Autodesk Fusion 360 part; units mm, degrees
(part 2 of 2)
sketch "Sketch5" plane through (0, 0, 32) normal (0, 0, 1) x (-1, 0, 0)
  line L0 (-236, -90) -> (0, -90)
  line L1 (0, -90) -> (0, -50)
  line L2 (0, -50) -> (-236, -50)
  line L3 (-236, -50) -> (-236, -90)
  line L4 (-4, -87) -> (-4, -53)
  line L5 (-108, -90) -> (-118, -90)
  line L6 (-4, -53) -> (-10, -53)
  line L7 (0, -90) -> (-10, -90)
  line L8 (0, -50) -> (0, -90)
  line L9 (-114, -87) -> (-114, -53)
  line L10 (0, -90) -> (-10, -90)
  line L11 (-118, -90) -> (-118, -50)
  line L12 (-10, -90) -> (-108, -90)
  line L13 (-10, -90) -> (-10, -50)
  line L14 (-108, -87) -> (-114, -87)
  line L15 (-4, -53) -> (-10, -53)
  line L16 (-10, -87) -> (-4, -87)
  line L17 (-10, -53) -> (-10, -87)
  line L18 (-108, -50) -> (-108, -90)
  line L19 (-10, -53) -> (-10, -87)
  line L20 (-118, -50) -> (-108, -50)
  line L21 (-108, -50) -> (-10, -50)
  line L22 (-10, -87) -> (-4, -87)
  line L23 (-108, -90) -> (-108, -50)
  line L24 (-114, -53) -> (-108, -53)
  line L25 (0, -50) -> (0, -90)
  line L26 (-10, -50) -> (0, -50)
  line L27 (-4, -87) -> (-4, -53)
  line L28 (-108, -53) -> (-108, -87)
  line L29 (-10, -50) -> (0, -50)
  line L30 (-10, -90) -> (-10, -50)
  line L31 (-10, -50) -> (-10, -90)
  line L32 (-122, -87) -> (-122, -53)
  line L33 (-226, -90) -> (-236, -90)
  line L34 (-122, -53) -> (-128, -53)
  line L35 (-118, -90) -> (-128, -90)
  line L36 (-118, -50) -> (-118, -90)
  line L37 (-232, -87) -> (-232, -53)
  line L38 (-118, -90) -> (-128, -90)
  line L39 (-236, -90) -> (-236, -50)
  line L40 (-128, -90) -> (-226, -90)
  line L41 (-128, -90) -> (-128, -50)
  line L42 (-226, -87) -> (-232, -87)
  line L43 (-122, -53) -> (-128, -53)
  line L44 (-128, -87) -> (-122, -87)
  line L45 (-128, -53) -> (-128, -87)
  line L46 (-226, -50) -> (-226, -90)
  line L47 (-128, -53) -> (-128, -87)
  line L48 (-236, -50) -> (-226, -50)
  line L49 (-226, -50) -> (-128, -50)
  line L50 (-128, -87) -> (-122, -87)
  line L51 (-226, -90) -> (-226, -50)
  line L52 (-232, -53) -> (-226, -53)
  line L53 (-118, -50) -> (-118, -90)
  line L54 (-128, -50) -> (-118, -50)
  line L55 (-122, -87) -> (-122, -53)
  line L56 (-226, -53) -> (-226, -87)
  line L57 (-128, -50) -> (-118, -50)
  line L58 (-128, -90) -> (-128, -50)
  line L59 (-128, -50) -> (-128, -90)
  line L60 (-4, -177) -> (-4, -143)
  line L61 (-108, -180) -> (-118, -180)
  line L62 (-4, -143) -> (-10, -143)
  line L63 (0, -180) -> (-10, -180)
  line L64 (0, -140) -> (0, -180)
  line L65 (-114, -177) -> (-114, -143)
  line L66 (0, -180) -> (-10, -180)
  line L67 (-118, -180) -> (-118, -140)
  line L68 (-10, -180) -> (-108, -180)
  line L69 (-10, -180) -> (-10, -140)
  line L70 (-108, -177) -> (-114, -177)
  line L71 (-4, -143) -> (-10, -143)
  line L72 (-10, -177) -> (-4, -177)
  line L73 (-10, -143) -> (-10, -177)
  line L74 (-108, -140) -> (-108, -180)
  line L75 (-10, -143) -> (-10, -177)
  line L76 (-118, -140) -> (-108, -140)
  line L77 (-108, -140) -> (-10, -140)
  line L78 (-10, -177) -> (-4, -177)
  line L79 (-108, -180) -> (-108, -140)
  line L80 (-114, -143) -> (-108, -143)
  line L81 (0, -140) -> (0, -180)
  line L82 (-10, -140) -> (0, -140)
  line L83 (-4, -177) -> (-4, -143)
  line L84 (-108, -143) -> (-108, -177)
  line L85 (-10, -140) -> (0, -140)
  line L86 (-10, -180) -> (-10, -140)
  line L87 (-10, -140) -> (-10, -180)
  line L88 (-122, -177) -> (-122, -143)
  line L89 (-226, -180) -> (-236, -180)
  line L90 (-122, -143) -> (-128, -143)
  line L91 (-118, -180) -> (-128, -180)
  line L92 (-118, -140) -> (-118, -180)
  line L93 (-232, -177) -> (-232, -143)
  line L94 (-118, -180) -> (-128, -180)
  line L95 (-236, -180) -> (-236, -140)
  line L96 (-128, -180) -> (-226, -180)
  line L97 (-128, -180) -> (-128, -140)
  line L98 (-226, -177) -> (-232, -177)
  line L99 (-122, -143) -> (-128, -143)
  line L100 (-128, -177) -> (-122, -177)
  line L101 (-128, -143) -> (-128, -177)
  line L102 (-226, -140) -> (-226, -180)
  line L103 (-128, -143) -> (-128, -177)
  line L104 (-236, -140) -> (-226, -140)
  line L105 (-226, -140) -> (-128, -140)
  line L106 (-128, -177) -> (-122, -177)
  line L107 (-226, -180) -> (-226, -140)
  line L108 (-232, -143) -> (-226, -143)
  line L109 (-118, -140) -> (-118, -180)
  line L110 (-128, -140) -> (-118, -140)
  line L111 (-122, -177) -> (-122, -143)
  line L112 (-226, -143) -> (-226, -177)
  line L113 (-128, -140) -> (-118, -140)
  line L114 (-128, -180) -> (-128, -140)
  line L115 (-128, -140) -> (-128, -180)
  line L116 (-4, -87) -> (-4, -53)
  line L117 (-108, -90) -> (-118, -90)
  line L118 (-4, -53) -> (-10, -53)
  line L119 (0, -90) -> (-10, -90)
  line L120 (0, -50) -> (0, -90)
  line L121 (-114, -87) -> (-114, -53)
  line L122 (0, -90) -> (-10, -90)
  line L123 (-118, -90) -> (-118, -50)
  line L124 (-10, -90) -> (-108, -90)
  line L125 (-10, -90) -> (-10, -50)
  line L126 (-108, -87) -> (-114, -87)
  line L127 (-4, -53) -> (-10, -53)
  line L128 (-10, -87) -> (-4, -87)
  line L129 (-10, -53) -> (-10, -87)
  line L130 (-108, -50) -> (-108, -90)
  line L131 (-10, -53) -> (-10, -87)
  line L132 (-118, -50) -> (-108, -50)
  line L133 (-108, -50) -> (-10, -50)
  line L134 (-10, -87) -> (-4, -87)
  line L135 (-108, -90) -> (-108, -50)
  line L136 (-114, -53) -> (-108, -53)
  line L137 (0, -50) -> (0, -90)
  line L138 (-10, -50) -> (0, -50)
  line L139 (-4, -87) -> (-4, -53)
  line L140 (-108, -53) -> (-108, -87)
  line L141 (-10, -50) -> (0, -50)
  line L142 (-10, -90) -> (-10, -50)
  line L143 (-10, -50) -> (-10, -90)
  line L144 (-128, -267) -> (-122, -267)
  line L145 (-10, -230) -> (0, -230)
  line L146 (0, -270) -> (-10, -270)
  line L147 (-128, -230) -> (-128, -270)
  line L148 (-118, -270) -> (-118, -230)
  line L149 (-226, -233) -> (-226, -267)
  line L150 (0, -230) -> (0, -270)
  line L151 (-108, -270) -> (-118, -270)
  line L152 (-118, -270) -> (-128, -270)
  line L153 (-226, -270) -> (-226, -230)
  line L154 (-118, -230) -> (-108, -230)
  line L155 (0, -230) -> (0, -270)
  line L156 (-128, -230) -> (-118, -230)
  line L157 (-10, -230) -> (-10, -270)
  line L158 (-118, -230) -> (-118, -270)
  line L159 (-10, -270) -> (-108, -270)
  line L160 (-10, -267) -> (-4, -267)
  line L161 (-10, -233) -> (-10, -267)
  line L162 (-128, -230) -> (-118, -230)
  line L163 (-10, -270) -> (-10, -230)
  line L164 (-236, -270) -> (-236, -230)
  line L165 (-128, -270) -> (-128, -230)
  line L166 (-122, -233) -> (-128, -233)
  line L167 (-10, -267) -> (-4, -267)
  line L168 (-122, -267) -> (-122, -233)
  line L169 (-10, -233) -> (-10, -267)
  line L170 (-10, -270) -> (-10, -230)
  line L171 (-236, -230) -> (-226, -230)
  line L172 (-128, -270) -> (-128, -230)
  line L173 (-128, -233) -> (-128, -267)
  line L174 (-226, -267) -> (-232, -267)
  line L175 (-108, -233) -> (-108, -267)
  line L176 (-128, -233) -> (-128, -267)
  line L177 (-122, -267) -> (-122, -233)
  line L178 (-118, -270) -> (-128, -270)
  line L179 (-226, -230) -> (-128, -230)
  line L180 (-4, -233) -> (-10, -233)
  line L181 (-10, -230) -> (0, -230)
  line L182 (-108, -230) -> (-10, -230)
  line L183 (-4, -233) -> (-10, -233)
  line L184 (0, -270) -> (-10, -270)
  line L185 (-108, -267) -> (-114, -267)
  line L186 (-128, -270) -> (-226, -270)
  line L187 (-4, -267) -> (-4, -233)
  line L188 (-128, -267) -> (-122, -267)
  line L189 (-114, -233) -> (-108, -233)
  line L190 (-232, -267) -> (-232, -233)
  line L191 (-114, -267) -> (-114, -233)
  line L192 (-226, -230) -> (-226, -270)
  line L193 (-232, -233) -> (-226, -233)
  line L194 (-108, -270) -> (-108, -230)
  line L195 (-226, -270) -> (-236, -270)
  line L196 (-122, -233) -> (-128, -233)
  line L197 (-108, -230) -> (-108, -270)
  line L198 (-4, -267) -> (-4, -233)
  line L199 (-118, -230) -> (-118, -270)
  dimension "d47" = 10
  dimension "d48" = 40
  dimension "d49" = 3
  dimension "d50" = 4
  dimension "d51" = 3
  dimension "d52" = 10
  dimension "d53" = 40
  dimension "d54" = 3
  dimension "d55" = 4
  dimension "d56" = 3
  dimension "d57" = 10
  dimension "d58" = 40
  dimension "d59" = 98
  dimension "d60" = 3
  dimension "d61" = 3
  dimension "d62" = 4
  dimension "d63" = 10
  dimension "d64" = 40
  dimension "d65" = 3
  dimension "d66" = 4
  dimension "d67" = 3
  dimension "d68" = 10
  dimension "d69" = 40
  dimension "d70" = 3
  dimension "d71" = 4
  dimension "d72" = 3
  dimension "d73" = 10
  dimension "d74" = 40
  dimension "d75" = 98
  dimension "d76" = 3
  dimension "d77" = 3
  dimension "d78" = 4
  dimension "d79" = 10
  dimension "d80" = 40
  dimension "d81" = 3
  dimension "d82" = 4
  dimension "d83" = 3
  dimension "d84" = 10
  dimension "d85" = 40
  dimension "d86" = 3
  dimension "d87" = 4
  dimension "d88" = 3
  dimension "d89" = 10
  dimension "d90" = 40
  dimension "d91" = 98
  dimension "d92" = 3
  dimension "d93" = 3
  dimension "d94" = 4
  dimension "d95" = 10
  dimension "d96" = 40
  dimension "d97" = 3
  dimension "d98" = 4
  dimension "d99" = 3
  dimension "d100" = 10
  dimension "d101" = 40
  dimension "d102" = 3
  dimension "d103" = 4
  dimension "d104" = 3
  dimension "d105" = 10
  dimension "d106" = 40
  dimension "d107" = 98
  dimension "d108" = 3
  dimension "d109" = 3
  dimension "d110" = 4
  dimension "d111" = 10
  dimension "d112" = 40
  dimension "d113" = 3
  dimension "d114" = 4
  dimension "d115" = 3
  dimension "d116" = 10
  dimension "d117" = 40
  dimension "d118" = 3
  dimension "d119" = 4
  dimension "d120" = 3
  dimension "d121" = 10
  dimension "d122" = 40
  dimension "d123" = 98
  dimension "d124" = 3
  dimension "d125" = 3
  dimension "d126" = 4
  dimension "d127" = 10
  dimension "d128" = 40
  dimension "d129" = 3
  dimension "d130" = 4
  dimension "d131" = 3
  dimension "d132" = 10
  dimension "d133" = 40
  dimension "d134" = 3
  dimension "d135" = 4
  dimension "d136" = 3
  dimension "d137" = 10
  dimension "d138" = 40
  dimension "d139" = 98
  dimension "d140" = 3
  dimension "d141" = 3
  dimension "d142" = 4
  dimension "d143" = 10
  dimension "d144" = 40
  dimension "d145" = 3
  dimension "d146" = 4
  dimension "d147" = 3
  dimension "d148" = 10
  dimension "d149" = 40
  dimension "d150" = 3
  dimension "d151" = 4
  dimension "d152" = 3
  dimension "d153" = 10
  dimension "d154" = 40
  dimension "d155" = 98
  dimension "d156" = 3
  dimension "d157" = 3
  dimension "d158" = 4
  constraint horizontal L10
  constraint vertical L13
  constraint horizontal L26
  constraint vertical L8
  constraint horizontal L22
  constraint vertical L4
  constraint horizontal L6
  constraint vertical L17
  constraint coincident L16.start L13
  constraint horizontal L7
  constraint vertical L30
  constraint horizontal L29
  constraint vertical L25
  constraint horizontal L16
  constraint vertical L27
  constraint horizontal L15
  constraint vertical L19
  constraint coincident L16.start L30
  constraint horizontal L5
  constraint vertical L11
  constraint horizontal L20
  constraint vertical L18
  constraint horizontal L14
  constraint vertical L9
  constraint horizontal L24
  constraint vertical L28
  constraint coincident L14.start L18
  constraint horizontal L12
  constraint vertical L23
  constraint horizontal L21
  constraint vertical L31
  constraint horizontal L38
  constraint vertical L41
  constraint horizontal L54
  constraint vertical L36
  constraint horizontal L50
  constraint vertical L32
  constraint horizontal L34
  constraint vertical L45
  constraint coincident L44.start L41
  constraint horizontal L35
  constraint vertical L58
  constraint horizontal L57
  constraint vertical L53
  constraint horizontal L44
  constraint vertical L55
  constraint horizontal L43
  constraint vertical L47
  constraint coincident L44.start L58
  constraint horizontal L33
  constraint vertical L39
  constraint horizontal L48
  constraint vertical L46
  constraint horizontal L42
  constraint vertical L37
  constraint horizontal L52
  constraint vertical L56
  constraint coincident L42.start L46
  constraint horizontal L40
  constraint vertical L51
  constraint horizontal L49
  constraint vertical L59
  constraint horizontal L66
  constraint vertical L69
  constraint horizontal L82
  constraint vertical L64
  constraint horizontal L78
  constraint vertical L60
  constraint horizontal L62
  constraint vertical L73
  constraint coincident L72.start L69
  constraint horizontal L63
  constraint vertical L86
  constraint horizontal L85
  constraint vertical L81
  constraint horizontal L72
  constraint vertical L83
  constraint horizontal L71
  constraint vertical L75
  constraint coincident L72.start L86
  constraint horizontal L61
  constraint vertical L67
  constraint horizontal L76
  constraint vertical L74
  constraint horizontal L70
  constraint vertical L65
  constraint horizontal L80
  constraint vertical L84
  constraint coincident L70.start L74
  constraint horizontal L68
  constraint vertical L79
  constraint horizontal L77
  constraint vertical L87
  constraint horizontal L94
  constraint vertical L97
  constraint horizontal L110
  constraint vertical L92
  constraint horizontal L106
  constraint vertical L88
  constraint horizontal L90
  constraint vertical L101
  constraint coincident L100.start L97
  constraint horizontal L91
  constraint vertical L114
  constraint horizontal L113
  constraint vertical L109
  constraint horizontal L100
  constraint vertical L111
  constraint horizontal L99
  constraint vertical L103
  constraint coincident L100.start L114
  constraint horizontal L89
  constraint vertical L95
  constraint horizontal L104
  constraint vertical L102
  constraint horizontal L98
  constraint vertical L93
  constraint horizontal L108
  constraint vertical L112
  constraint coincident L98.start L102
  constraint horizontal L96
  constraint vertical L107
  constraint horizontal L105
  constraint vertical L115
  constraint horizontal L122
  constraint vertical L125
  constraint horizontal L138
  constraint vertical L120
  constraint horizontal L134
  constraint vertical L116
  constraint horizontal L118
  constraint vertical L129
  constraint coincident L16.start L125
  constraint horizontal L119
  constraint vertical L142
  constraint horizontal L141
  constraint vertical L137
  constraint horizontal L128
  constraint vertical L139
  constraint horizontal L127
  constraint vertical L131
  constraint coincident L16.start L142
  constraint horizontal L117
  constraint vertical L123
  constraint horizontal L132
  constraint vertical L130
  constraint horizontal L126
  constraint vertical L121
  constraint horizontal L136
  constraint vertical L140
  constraint coincident L14.start L130
  constraint horizontal L124
  constraint vertical L135
  constraint horizontal L133
  constraint vertical L143
  constraint horizontal L184
  constraint vertical L163
  constraint horizontal L145
  constraint vertical L155
  constraint horizontal L160
  constraint vertical L187
  constraint horizontal L180
  constraint vertical L161
  constraint coincident L160.start L163
  constraint horizontal L146
  constraint vertical L170
  constraint horizontal L181
  constraint vertical L150
  constraint horizontal L167
  constraint vertical L198
  constraint horizontal L183
  constraint vertical L169
  constraint coincident L160.start L170
  constraint horizontal L151
  constraint vertical L148
  constraint horizontal L154
  constraint vertical L197
  constraint horizontal L185
  constraint vertical L191
  constraint horizontal L189
  constraint vertical L175
  constraint coincident L175.end L197
  constraint horizontal L159
  constraint vertical L194
  constraint horizontal L182
  constraint vertical L157
  constraint horizontal L178
  constraint vertical L165
  constraint horizontal L162
  constraint vertical L158
  constraint horizontal L188
  constraint vertical L168
  constraint horizontal L196
  constraint vertical L176
  constraint coincident L144.start L165
  constraint horizontal L152
  constraint vertical L172
  constraint horizontal L156
  constraint vertical L199
  constraint horizontal L144
  constraint vertical L177
  constraint horizontal L166
  constraint vertical L173
  constraint coincident L144.start L172
  constraint horizontal L195
  constraint vertical L164
  constraint horizontal L171
  constraint vertical L192
  constraint horizontal L174
  constraint vertical L190
  constraint horizontal L193
  constraint vertical L149
  constraint coincident L149.end L192
  constraint horizontal L186
  constraint vertical L153
  constraint horizontal L179
  constraint vertical L147
  measures "d47" distance of L0.end L7.end
  measures "d48" distance of L1.end L0.end
  measures "d49" distance of L10 L22
  measures "d50" distance of L4 L8
  measures "d51" distance of L6 L26
  measures "d52" distance of L7.end L0.end
  measures "d53" distance of L0.end L1.end
  measures "d54" distance of L7 L16
  measures "d55" distance of L25 L27
  measures "d56" distance of L15 L29
  measures "d57" distance of L5.start L5.end
  measures "d58" distance of L5.start L18.start
  measures "d59" distance of L18 L30
  measures "d60" distance of L5 L14
  measures "d61" distance of L20 L24
  measures "d62" distance of L9 L11
  measures "d63" distance of L5.end L35.end
  measures "d64" distance of L11.end L5.end
  measures "d65" distance of L38 L50
  measures "d66" distance of L32 L36
  measures "d67" distance of L34 L54
  measures "d68" distance of L35.end L5.end
  measures "d69" distance of L5.end L11.end
  measures "d70" distance of L35 L44
  measures "d71" distance of L53 L55
  measures "d72" distance of L43 L57
  measures "d73" distance of L33.start L0.start
  measures "d74" distance of L33.start L46.start
  measures "d75" distance of L46 L58
  measures "d76" distance of L33 L42
  measures "d77" distance of L48 L52
  measures "d78" distance of L37 L39
  measures "d79" distance of L63.start L63.end
  measures "d80" distance of L64.start L63.start
  measures "d81" distance of L66 L78
  measures "d82" distance of L60 L64
  measures "d83" distance of L62 L82
  measures "d84" distance of L63.end L63.start
  measures "d85" distance of L63.start L64.start
  measures "d86" distance of L63 L72
  measures "d87" distance of L81 L83
  measures "d88" distance of L71 L85
  measures "d89" distance of L61.start L61.end
  measures "d90" distance of L61.start L74.start
  measures "d91" distance of L74 L86
  measures "d92" distance of L61 L70
  measures "d93" distance of L76 L80
  measures "d94" distance of L65 L67
  measures "d95" distance of L61.end L91.end
  measures "d96" distance of L67.end L61.end
  measures "d97" distance of L94 L106
  measures "d98" distance of L88 L92
  measures "d99" distance of L90 L110
  measures "d100" distance of L91.end L61.end
  measures "d101" distance of L61.end L67.end
  measures "d102" distance of L91 L100
  measures "d103" distance of L109 L111
  measures "d104" distance of L99 L113
  measures "d105" distance of L89.start L89.end
  measures "d106" distance of L89.start L102.start
  measures "d107" distance of L102 L114
  measures "d108" distance of L89 L98
  measures "d109" distance of L104 L108
  measures "d110" distance of L93 L95
  measures "d111" distance of L0.end L7.end
  measures "d112" distance of L1.end L0.end
  measures "d113" distance of L122 L134
  measures "d114" distance of L116 L120
  measures "d115" distance of L118 L138
  measures "d116" distance of L7.end L0.end
  measures "d117" distance of L0.end L1.end
  measures "d118" distance of L119 L128
  measures "d119" distance of L137 L139
  measures "d120" distance of L127 L141
  measures "d121" distance of L5.start L5.end
  measures "d122" distance of L5.start L18.start
  measures "d123" distance of L130 L142
  measures "d124" distance of L117 L126
  measures "d125" distance of L132 L136
  measures "d126" distance of L121 L123
  measures "d127" distance of L146.start L146.end
  measures "d128" distance of L145.end L146.start
  measures "d129" distance of L160 L184
  measures "d130" distance of L155 L187
  measures "d131" distance of L145 L180
  measures "d132" distance of L146.end L146.start
  measures "d133" distance of L146.start L145.end
  measures "d134" distance of L146 L167
  measures "d135" distance of L150 L198
  measures "d136" distance of L181 L183
  measures "d137" distance of L151.start L148.start
  measures "d138" distance of L154.end L151.start
  measures "d139" distance of L170 L197
  measures "d140" distance of L151 L185
  measures "d141" distance of L154 L189
  measures "d142" distance of L148 L191
  measures "d143" distance of L147.end L148.start
  measures "d144" distance of L148.start L148.end
  measures "d145" distance of L178 L188
  measures "d146" distance of L158 L168
  measures "d147" distance of L162 L196
  measures "d148" distance of L148.start L147.end
  measures "d149" distance of L148.end L148.start
  measures "d150" distance of L144 L152
  measures "d151" distance of L177 L199
  measures "d152" distance of L156 L166
  measures "d153" distance of L164.start L153.start
  measures "d154" distance of L153.end L153.start
  measures "d155" distance of L172 L192
  measures "d156" distance of L174 L195
  measures "d157" distance of L171 L193
  measures "d158" distance of L164 L190
extrude "Extrude4" cut sketch "Sketch4" sketch "Sketch5" against normal blind 2 contours L21 L24 L25 L26 L27 L28 L30 L32 L34 L35 L47 of sketch 2 contours L0 L2 L40 L41 L45 L46 L47 L49 L51 L56 L58 L59 | L37 L42 L46 L51 L52 L56 | L32 L34 L41 L43 L44 L45 L47 L50 L55 L58 L59 | L0 L2 L12 L13 L17 L18 L19 L21 L23 L28 L30 L31 L124 L125 L129 L130 L131 L133 L135 L140 L142 L143 | L9 L14 L18 L23 L24 L28 L121 L126 L130 L135 L136 L140 | L60 L62 L69 L71 L72 L73 L75 L78 L83 L86 L87 | L68 L69 L73 L74 L75 L77 L79 L84 L86 L87 | L65 L70 L74 L79 L80 L84 | L96 L97 L101 L102 L103 L105 L107 L112 L114 L115 | L88 L90 L97 L99 L100 L101 L103 L106 L111 L114 L115 | L93 L98 L102 L107 L108 L112 | L144 L147 L165 L166 L168 L172 L173 L176 L177 L188 L196 | L147 L149 L153 L165 L172 L173 L176 L179 L186 L192 | L157 L159 L161 L163 L169 L170 L175 L182 L194 L197 | L149 L153 L174 L190 L192 L193 | L175 L185 L189 L191 L194 L197 | L157 L160 L161 L163 L167 L169 L170 L180 L183 L187 L198
sketch "Sketch6" plane through (0, 0, 30) normal (0, 0, 1) x (-1, 0, 0)
  line L0 (-128, -87) -> (-122, -87)
  line L1 (-122, -87) -> (-122, -53)
  line L2 (-122, -53) -> (-128, -53)
  line L3 (-128, -53) -> (-128, -50)
  line L4 (-128, -50) -> (-226, -50)
  line L5 (-226, -50) -> (-226, -53)
  line L6 (-226, -53) -> (-232, -53)
  line L7 (-232, -53) -> (-232, -87)
  line L8 (-232, -87) -> (-226, -87)
  line L9 (-226, -87) -> (-226, -90)
  line L10 (-226, -90) -> (-128, -90)
  line L11 (-128, -90) -> (-128, -87)
  line L12 (-128, -90) -> (-226, -90)
  line L13 (-226, -90) -> (-226, -50)
  line L14 (-226, -50) -> (-128, -50)
  line L15 (-128, -50) -> (-128, -90)
  line L16 (-108, -50) -> (-10, -50)
  line L17 (-10, -50) -> (-10, -90)
  line L18 (-10, -90) -> (-108, -90)
  line L19 (-108, -90) -> (-108, -50)
  line L20 (-10, -140) -> (-108, -140)
  line L21 (-108, -140) -> (-108, -180)
  line L22 (-108, -180) -> (-10, -180)
  line L23 (-10, -180) -> (-10, -140)
  line L24 (-128, -180) -> (-226, -180)
  line L25 (-226, -180) -> (-226, -140)
  line L26 (-226, -140) -> (-128, -140)
  line L27 (-128, -140) -> (-128, -180)
  line L28 (-128, -270) -> (-226, -270)
  line L29 (-226, -270) -> (-226, -230)
  line L30 (-226, -230) -> (-128, -230)
  line L31 (-128, -230) -> (-128, -270)
  line L32 (-10, -270) -> (-108, -270)
  line L33 (-108, -270) -> (-108, -230)
  line L34 (-108, -230) -> (-10, -230)
  line L35 (-10, -230) -> (-10, -270)
  constraint horizontal L12
  constraint vertical L13
  constraint horizontal L14
  constraint vertical L15
  constraint coincident L4.end L5.start
  constraint coincident L10.end L11.start
  constraint horizontal L16
  constraint vertical L17
  constraint horizontal L18
  constraint vertical L19
  constraint horizontal L20
  constraint vertical L21
  constraint horizontal L22
  constraint vertical L23
  constraint horizontal L24
  constraint vertical L25
  constraint horizontal L26
  constraint vertical L27
  constraint horizontal L28
  constraint vertical L29
  constraint horizontal L30
  constraint vertical L31
  constraint horizontal L32
  constraint vertical L33
  constraint horizontal L34
  constraint vertical L35
extrude "Extrude5" cut sketch "Sketch6" against normal blind 20 contours L3 L4 L5 L9 L10 L11 L12 L13 L14 L15 | L16 L17 L18 L19 | L20 L21 L22 L23 | L24 L25 L26 L27 | L28 L29 L30 L31 | L32 L33 L34 L35
extrude "Extrude6" add 9 faces at (1.3333, 64.3333, 32) (119.3333, 75.6667, 32) (234.6667, 64.3333, 32) (234.6667, 154.3333, 32) (119.3333, 165.6667, 32) (1.3333, 154.3333, 32) (1.3333, 244.3333, 32) (119.3333, 255.6667, 32) (234.6667, 244.3333, 32) along direction (0, 0, 1) blind 2
extrude "Extrude7" add 12 faces at (8, 255.6667, 30) (112, 244.3333, 30) (124, 255.6667, 30) (126, 165.6667, 30) (112, 154.3333, 30) (8, 154.3333, 30) (8, 64.3333, 30) (112, 64.3333, 30) (126, 64.3333, 30) (228, 64.3333, 30) (230, 165.6667, 30) (230, 244.3333, 30) along direction (0, 0, 1) blind 2

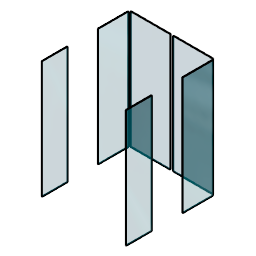
design "panels_lift"
part number: 2025-09-29-16-30-13-103
Autodesk Fusion 360 part; units mm, degrees
sketch "Sketch2" plane through (0, 0, 0) normal (0, 0, 1) x (1, 0, 0)
  circle A0 centre (369.0335, 129.9822) radius 9.5683
  line L0 (379, 0) -> (0, 0)
  circle A1 centre (9.9323, 390.2005) radius 9.8463
  circle A2 centre (369.0335, 9.9664) radius 9.58
  line L1 (0, 0) -> (0, 400)
  line L2 (379, 400) -> (379, 0)
  circle A3 centre (368.8758, 249.998) radius 10.0154
  circle A4 centre (357, 189.5) radius 10
  circle A5 centre (10, 130) radius 9.1446
  circle A6 centre (189.404, 390.0428) radius 10.4671
  circle A7 centre (21.6223, 189.5) radius 10
  line L3 (379, 400) -> (0, 400)
  line L4 (0, 400) -> (379, 400)
  line L5 (379, 0) -> (379, 400)
  line L6 (0, 0) -> (379, 0)
  circle A8 centre (10, 10) radius 9.64
  circle A9 centre (369.0335, 390.0428) radius 9.9043
  circle A10 centre (9.7746, 249.8403) radius 9.7282
  line L7 (0, 400) -> (0, 0)
  line L8 (12.0242, 16.0517) -> (8.0242, 16.0517)
  line L9 (8.0242, 16.0517) -> (8.0242, 126.0517)
  line L10 (8.0242, 126.0517) -> (12.0242, 126.0517)
  line L11 (12.0242, 126.0517) -> (12.0242, 16.0517)
  line L12 (371.1039, 14.7178) -> (367.1039, 14.7178)
  line L13 (367.1039, 14.7178) -> (367.1039, 124.7178)
  line L14 (371.1039, 124.7178) -> (371.1039, 14.7178)
  line L15 (367.1039, 124.7178) -> (371.1039, 124.7178)
  line L16 (367.0354, 385.2556) -> (371.0354, 385.2556)
  line L17 (371.0354, 385.2556) -> (371.0354, 255.2556)
  line L18 (371.0354, 255.2556) -> (367.0354, 255.2556)
  line L19 (367.0354, 255.2556) -> (367.0354, 385.2556)
  line L20 (11.9656, 254.7418) -> (7.9656, 254.7418)
  line L21 (7.9656, 384.7418) -> (11.9656, 384.7418)
  line L22 (7.9656, 254.7418) -> (7.9656, 384.7418)
  line L23 (11.9656, 384.7418) -> (11.9656, 254.7418)
  line L24 (14.078, 391.8365) -> (184.078, 391.8365)
  line L25 (184.078, 391.8365) -> (184.078, 387.8365)
  line L26 (184.078, 387.8365) -> (14.078, 387.8365)
  line L27 (14.078, 387.8365) -> (14.078, 391.8365)
  line L28 (364.6598, 392.0078) -> (364.6598, 388.0078)
  line L29 (194.6598, 392.0078) -> (364.6598, 392.0078)
  line L30 (364.6598, 388.0078) -> (194.6598, 388.0078)
  line L31 (194.6598, 388.0078) -> (194.6598, 392.0078)
  dimension "d21" = 4
  dimension "d22" = 110
  dimension "d23" = 4
  dimension "d24" = 110
  dimension "d25" = 4
  dimension "d26" = 130
  dimension "d27" = 4
  dimension "d28" = 130
  dimension "d29" = 170
  dimension "d30" = 4
  dimension "d31" = 170
  dimension "d32" = 4
  constraint horizontal L0
  constraint vertical L1
  constraint horizontal L4
  constraint vertical L2
  constraint coincident L1.end L3.end
  constraint coincident L0.start L2.end
  constraint horizontal L8
  constraint vertical L9
  constraint horizontal L10
  constraint vertical L11
  constraint horizontal L12
  constraint vertical L13
  constraint horizontal L15
  constraint vertical L14
  constraint horizontal L16
  constraint vertical L17
  constraint horizontal L18
  constraint vertical L19
  constraint horizontal L21
  constraint vertical L23
  constraint horizontal L20
  constraint vertical L22
  constraint horizontal L24
  constraint vertical L25
  constraint horizontal L26
  constraint vertical L27
  constraint horizontal L29
  constraint vertical L28
  constraint horizontal L30
  constraint vertical L31
  measures "d21" distance of L8.start L8.end
  measures "d22" distance of L8.start L10.end
  measures "d23" distance of L12.start L12.end
  measures "d24" distance of L12.start L14.start
  measures "d25" distance of L16.start L16.end
  measures "d26" distance of L16.start L18.end
  measures "d27" distance of L21.end L21.start
  measures "d28" distance of L20.end L21.start
  measures "d29" distance of L24.start L24.end
  measures "d30" distance of L24.start L26.end
  measures "d31" distance of L29.start L28.start
  measures "d32" distance of L29.start L30.end
extrude "Extrude2" add sketch "Sketch2" along normal blind 500 contours A0 L13 L14 L15 | A0 A2 L13 L14 | A2 L12 L13 L14 | A6 A9 L29 L30 | A6 L29 L30 L31 | A1 L21 L22 L23 | A1 A10 L22 L23 | A9 L28 L29 L30 | A6 L24 L25 L26 | A1 A6 L24 L26 | A1 L24 L26 L27 | A10 L20 L22 L23 | A3 A9 L17 L19 | A9 L16 L17 L19 | A3 L17 L18 L19 | A5 L9 L10 L11 | A5 A8 L9 L11 | A8 L8 L9 L11 picked at (369.3281, 123.2928) picked at (369.3281, 16.3177) picked at (10.1905, 256.3379) picked at (369.26, 256.8299) picked at (10.2482, 124.3284) picked at (10.248, 17.2394) makes body 1 at (371.0354, 341.9222, 166.6667) makes body 2 at (7.9656, 298.0752, 166.6667) makes body 3 at (367.1039, 51.3845, 166.6667) makes body 4 at (251.3264, 392.0078, 166.6667) makes body 5 at (70.7447, 391.8365, 166.6667) makes body 6 at (8.0242, 52.7184, 166.6667)
